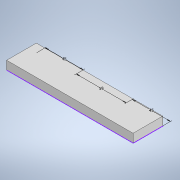
# Autodesk Inventor part: kill swich tampa
Saved by Autodesk Inventor 2022 (Build 260153000, 153)
## iProperties
Created: 2022-03-09
Part Number: kill swich tampa
Material: Genérico
Document SubType Name: Modeling
Designer: Guilherme
Density: 1 g/cm^3
Appearance: Padrão
Author: Guilherme
Autodesk Inventor part; units mm, degrees
ref_plane "YZ Plane" through (0, 0, 0) normal (1, 0, 0) x (0, 1, 0)
ref_plane "XZ Plane" through (0, 0, 0) normal (0, 1, 0) x (-1, 0, 0)
ref_plane "XY Plane" through (0, 0, 0) normal (0, 0, 1) x (1, 0, 0)
sketch "Esboço1" plane through (0, 0, 0) normal (0, 1, 0) x (-1, 0, 0)
  line L0 (29.5, 17.5) -> (-29.5, 17.5)
  line L1 (-29.5, 17.5) -> (-29.5, -17.5)
  line L2 (-29.5, -17.5) -> (29.5, -17.5)
  line L3 (29.5, -17.5) -> (29.5, 17.5)
  line L4 (29.5, 17.5) -> (-29.5, -17.5) construction
  line L5 (-29.5, 17.5) -> (29.5, -17.5) construction
  line L6 (29.5, 17.5) -> (74.5, 17.5)
  line L7 (74.5, 17.5) -> (74.5, -17.5)
  line L8 (74.5, -17.5) -> (29.5, -17.5)
  line L9 (29.5, -17.5) -> (29.5, 17.5)
  line L10 (-29.5, -17.5) -> (-29.5, 17.5)
  line L11 (-29.5, 17.5) -> (-74.5, 17.5)
  line L12 (-74.5, 17.5) -> (-74.5, -17.5)
  line L13 (-74.5, -17.5) -> (-29.5, -17.5)
  line L14 (-29.5, -17.5) -> (-29.5, 17.5)
  point P0 (0, 0)
  dimension "d0" = 59
  dimension "d2" = 45
  dimension "d4" = 45
  constraints: 30 end point, 6 parallel, 3 horizontal, 3 perpendicular, 2 midpoint, 1 point on line
  measures "d0" distance of L2.end L1.end
  measures "d2" distance of L7.end L8.end
  measures "d4" distance of L13.end L12.end
extrude "Extrusão1" add sketch "Esboço1" along normal blind 10
